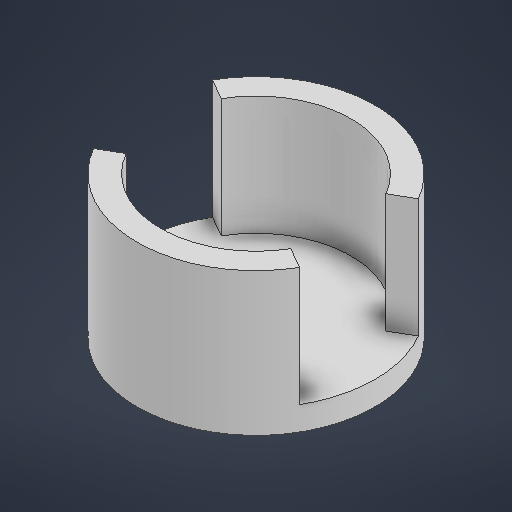
# Autodesk Inventor part: rotacniZaklad
Saved by Autodesk Inventor 2026 (Build 300175000, 175)
## iProperties
Created: 2025-04-11
Part Number: rotacniZaklad
Material: Generic
Document SubType Name: Modeling
Designer: vitgr
Density: 1 g/cm^3
Appearance: Default
Author: vitgr
Autodesk Inventor part; units mm, degrees
ref_plane "YZ Plane" through (0, 0, 0) normal (1, 0, 0) x (0, 1, 0)
ref_plane "XZ Plane" through (0, 0, 0) normal (0, 1, 0) x (-1, 0, 0)
ref_plane "XY Plane" through (0, 0, 0) normal (0, 0, 1) x (1, 0, 0)
sketch "Sketch1" plane through (0, 0, 0) normal (0, 1, 0) x (-1, 0, 0)
  line L0 (17.3205, -10) -> (21.6506, -12.5)
  line L1 (0, 0) -> (25, 0) construction
  line L2 (17.3205, 10) -> (21.6506, 12.5)
  line L3 (-17.3205, -10) -> (-21.6506, -12.5)
  line L4 (-17.3205, 10) -> (-21.6506, 12.5)
  arc A0 (17.3205, 10) -> (-17.3205, 10) centre (0, 0) ccw
  arc A1 (-17.3205, -10) -> (17.3205, -10) centre (0, 0) ccw
  arc A2 (21.6506, 12.5) -> (-21.6506, 12.5) centre (0, 0) ccw
  arc A3 (-21.6506, -12.5) -> (21.6506, -12.5) centre (0, 0) ccw
  circle A4 centre (0, 0) radius 25
  point P0 (0, 20)
  point P1 (0, -20)
  dimension "d13" = 50
  dimension "d4" = 30
  dimension "d10" = 40
  dimension "d11" = 20
  constraints: 10 end point, 10 point on circle, 4 centre point, 2 coincident, 1 horizontal, 1 symmetric about line, 3 other
  measures "d4" angle of L0 L1
  measures "d10" distance of point (0, 20) point (0, -20)
  measures "d11" radius of A1
sketch "Sketch2" plane through (0, 0, 0) normal (0, 1, 0) x (-1, 0, 0)
  circle A0 centre (0, 0) radius 25
  dimension "d14" = 50
  constraints: 1 centre point, 1 coincident
  measures "d14" diameter of A0
extrude "Extrusion1" add sketch "Sketch2" against normal blind 5
extrude "Extrusion2" add sketch "Sketch1" along normal blind 25 contours L0 A3 L3 A1 | A2 L2 A0 L4
body "Solid1"
